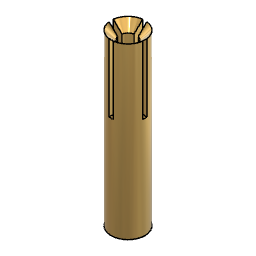
electrode puck v2 contact plug v5 (Autodesk Fusion 360 design; units mm, degrees)
Autodesk Fusion 360 part; units mm, degrees
cylinder "CylinderPrimitive1" add diameter 2 height 10 placed x (1, 0, 0) y (0, 0, -1) z (0, 1, 0) at (0, 0, 0)
hole "Hole1" at (0, 10, 0) direction (0, -1, 0) diameter 1 depth 4 tip angle 118
hole "Hole2" at (0, 0, 0) direction (0, 1, 0) diameter 1.5 depth 4 tip angle 118
chamfer "Chamfer1" distance 0.5 angle 45 1 edges at (0.1808, 10, -0.4662) measured on face at (0.8291, 10, 0.0621)
sketch "Sketch2" plane through (0, 0, 0) normal (1, 0, 0) x (0, 0, -1)
  line L0 (-2.7313, 12.0493) -> (-0.0081, 12.0493)
  line L1 (-0.0081, 12.0493) -> (-0.0081, 6)
  line L2 (-0.0081, 6) -> (-2.7313, 6)
  line L3 (-2.7313, 6) -> (-2.7313, 12.0493)
  line L4 (1, 10) -> (-1, 10)
  dimension "d15" = 4
  constraint horizontal L0
  constraint vertical L1
  constraint horizontal L2
  constraint vertical L3
  measures "d15" distance of L2 L4
extrude "Extrude1" cut sketch "Sketch2" along normal mid plane 0.25
pattern_circular "C-Pattern1" count 4 over 360 about axis through (0, 1.75, 0) along (0, 1, 0) of "Extrude1"
